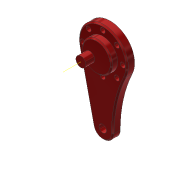
# Autodesk Inventor part: COXA_ROLL_SERVO-OUTPUT
Saved by Autodesk Inventor 2019.4 (Build 234330000, 330)
## iProperties
Created: 2019-10-21
Part Number: COXA_ROLL_SERVO-OUTPUT
Material: 一般
Document SubType Name: Modeling
Designer: y6tada
Density: 1 g/cm^3
Appearance: 滑らか - 赤
Author: y6tada
Autodesk Inventor part; units mm, degrees
ref_plane "YZ Plane" through (0, 0, 0) normal (1, 0, 0) x (0, 1, 0)
ref_plane "XZ Plane" through (0, 0, 0) normal (0, 1, 0) x (-1, 0, 0)
ref_plane "XY Plane" through (0, 0, 0) normal (0, 0, 1) x (1, 0, 0)
sketch "スケッチ1" plane through (0, 0, 0) normal (0, 0, 1) x (1, 0, 0)
  line L0 (0, 0) -> (-2.7189, -1.2679) construction
  line L1 (0, 0) -> (0, -26) construction
  arc A0 (8.8407, -4.1114) -> (-9.5086, -2.1563) centre (0, 0) ccw
  arc A1 (-3.901, -26.8846) -> (4, -26) centre (0, -26) ccw
  arc A2 (8.8407, -4.1114) -> (4, -26) centre (55.9076, -26) ccw
  line L2 (-9.5086, -2.1563) -> (-3.901, -26.8846)
  line L3 (0, -26) -> (4, -26) construction
  circle A3 centre (0, 0) radius 8 construction
  point P0 (8, 0)
  point P1 (5.6569, 5.6569)
  point P2 (0, 8)
  point P3 (-5.6569, 5.6569)
  point P4 (-8, 0)
  point P5 (-5.6569, -5.6569)
  point P6 (0, -8)
  point P7 (5.6569, -5.6569)
  point P8 (0, -26)
  dimension "d38" = 16
  dimension "d2" = 3
  dimension "d4" = 26
  dimension "d6" = 9.75
  dimension "d7" = 4
  dimension "d11" = 360
  dimension "d37" = 65
  constraints: 8 end point, 6 point on circle, 5 coincident, 4 tangent, 3 centre point, 1 perpendicular, 1 point on line, 1 vertical, 1 vertical alignment, 11 other
  measures "d2" distance of L0.start L0.end
  measures "d4" distance of L0.start L1.end
  measures "d6" radius of A0
  measures "d7" radius of A1
  measures "d37" angle of L1 L0
extrude "押し出し1" add sketch "スケッチ1" along normal blind 3
sketch "スケッチ5" plane through (0, 0, 3) normal (0, 0, 1) x (1, 0, 0)
  circle A0 centre (0, 0) radius 6
  arc A1 (8.8407, -4.1114) -> (-9.5086, -2.1563) centre (0, 0) ccw construction
  dimension "d41" = 12
  constraints: 1 centre point, 1 coincident
  measures "d41" diameter of A0
extrude "押し出し4" add sketch "スケッチ5" along normal blind 2.5
hole "穴1" at (8, 0, 0) at (5.6569, 5.6569, 0) at (0, 8, 0) at (-5.6569, 5.6569, 0) at (-8, 0, 0) at (-5.6569, -5.6569, 0) at (0, -8, 0) at (5.6569, -5.6569, 0) direction (0, 0, 1) diameter 2 end through all
hole "穴2" at (0, -26, 0) direction (0, 0, 1) diameter 3 end through all
sketch "スケッチ2" plane through (0, 0, 0) normal (0, 0, -1) x (-1, 0, 0)
  circle A0 centre (0, 0) radius 4
  dimension "d30" = 8
  constraints: 1 centre point, 1 coincident
  measures "d30" diameter of A0
extrude "押し出し2" cut sketch "スケッチ2" against normal blind 2
sketch "スケッチ3" plane through (0, 0, 5.5) normal (0, 0, 1) x (1, 0, 0)
  circle A0 centre (-2.7189, -1.2679) radius 2
  point P0 (0, 0)
  dimension "d33" = 4
  constraints: 1 centre point, 1 coincident
  measures "d33" diameter of A0
extrude "押し出し3" add sketch "スケッチ3" along normal blind 3.2
chamfer "面取り1" distance 0.5 angle 45 5 edges at (-6, 0, 5.5) (1.033, 9.6951, 3) (-6.7048, -14.5204, 3) (0.4451, -29.9752, 3) (5.2246, -14.7913, 3)
